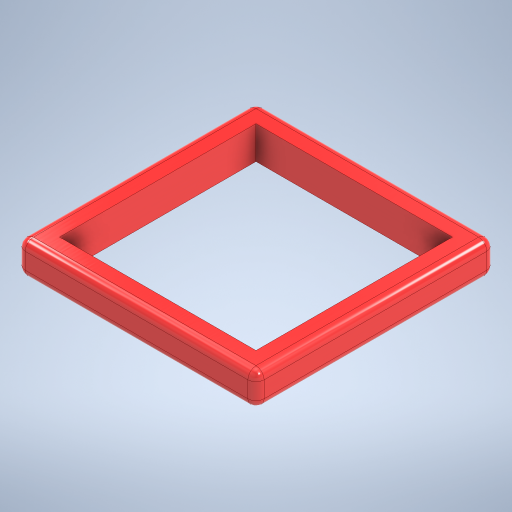
# Autodesk Inventor part: swerve red bumper
Saved by Autodesk Inventor 2023 (Build 270158030, 158C)
## iProperties
Created: 2022-07-20
Part Number: swerve red bumper
Material: Generic
Document SubType Name: Modeling
Designer: rm0990889
Density: 1 g/cm^3
Appearance: Light Red
Author: rm0990889
Autodesk Inventor part; units mm, degrees
ref_plane "YZ Plane" through (0, 0, 0) normal (1, 0, 0) x (0, 1, 0)
ref_plane "XZ Plane" through (0, 0, 0) normal (0, 1, 0) x (-1, 0, 0)
ref_plane "XY Plane" through (0, 0, 0) normal (0, 0, 1) x (1, 0, 0)
sketch "Sketch1" plane through (0, 0, 0) normal (0, 1, 0) x (-1, 0, 0)
  line L0 (9.3614, 10.2148) -> (-752.2576, 10.2148)
  line L1 (-752.2576, 10.2148) -> (-752.2576, -751.4042)
  line L2 (-752.2576, -751.4042) -> (9.3614, -751.4042)
  line L3 (9.3614, -751.4042) -> (9.3614, 10.2148)
  line L4 (91.9114, 92.7648) -> (-834.8076, 92.7648)
  line L5 (-834.8076, 92.7648) -> (-834.8076, -833.9542)
  line L6 (-834.8076, -833.9542) -> (91.9114, -833.9542)
  line L7 (91.9114, -833.9542) -> (91.9114, 92.7648)
  point P0 (0, 0)
  dimension "d0" = 761.619
  dimension "d1" = 761.619
  dimension "d2" = 82.55
  constraints: 16 end point, 4 parallel, 2 perpendicular, 1 horizontal, 3 other
  measures "d0" distance of L2.end L1.end
  measures "d1" distance of L1.end L0.end
  measures "d2" distance between parallel lines of L3 L7
extrude "Extrusion1" add sketch "Sketch1" along normal blind 127
fillet "Fillet1" radius 31.75 12 edges at (371.4481, 127, 92.7648) (834.8076, 127, -370.5947) (834.8076, 0, -370.5947) (371.4481, 0, 92.7648) (834.8076, 63.5, 92.7648) (371.4481, 127, -833.9542) (371.4481, 0, -833.9542) (834.8076, 63.5, -833.9542) (-91.9114, 63.5, -833.9542) (-91.9114, 127, -370.5947) (-91.9114, 63.5, 92.7648) (-91.9114, 0, -370.5947)
body "Solid1"
